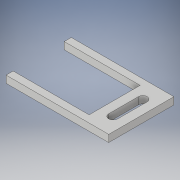
# Autodesk Inventor part: FixScan
Saved by Autodesk Inventor 2017 (Build 210142000, 142)
## iProperties
Part Number: FixScan
Material: Типовые
Document SubType Name: Modeling
Designer: yulia_000
Density: 1 g/cm^3
Appearance: По умолчанию
Author: yulia_000
Autodesk Inventor part; units mm, degrees
ref_plane "YZ Plane" through (0, 0, 0) normal (1, 0, 0) x (0, 1, 0)
ref_plane "XZ Plane" through (0, 0, 0) normal (0, 1, 0) x (-1, 0, 0)
ref_plane "XY Plane" through (0, 0, 0) normal (0, 0, 1) x (1, 0, 0)
sketch "Эскиз1" plane through (0, 0, 0) normal (0, 1, 0) x (-1, 0, 0)
  line L0 (0, 0) -> (9, 0)
  line L1 (9, 0) -> (9, -2.4)
  line L2 (9, -22) -> (0, -22)
  line L3 (0, -22) -> (0, 0)
  line L4 (9, -22) -> (34.6, -22)
  line L5 (34.6, -22) -> (34.6, -19.6)
  line L6 (34.6, -19.6) -> (9, -19.6)
  line L7 (9, -11) -> (0, -11)
  line L8 (9, 0) -> (34.6, 0)
  line L9 (34.6, 0) -> (34.6, -2.4)
  line L10 (34.6, -2.4) -> (9, -2.4)
  line L11 (9, -2.4) -> (9, -22)
  line L12 (4.5, -6) -> (4.5, -16) construction
  line L13 (3, -6) -> (3, -16)
  line L14 (6, -16) -> (6, -6)
  arc A0 (6, -6) -> (3, -6) centre (4.5, -6) ccw
  arc A1 (3, -16) -> (6, -16) centre (4.5, -16) ccw
  point P0 (4.5, -11)
  dimension "d0" = 9
  dimension "d1" = 22
  dimension "d2" = 25.6
  dimension "d3" = 2.4
  dimension "d4" = 5
  dimension "d5" = 3
  dimension "d6" = 30.1
  constraints: 32 end point, 4 parallel, 4 perpendicular, 4 point on circle, 4 tangent, 3 midpoint, 3 symmetric about line, 2 centre point, 2 horizontal, 2 point on line, 2 vertical
  measures "d0" distance of L2.start L2.end
  measures "d1" distance of L2.end L0.start
  measures "d2" distance of L2.start L4.end
  measures "d3" distance of L4.end L5.end
  measures "d4" distance of point (4.5, -11) L12.end
  measures "d5" diameter of A1
  measures "d6" distance between parallel lines of L5 L12
extrude "Выдавливание1" add sketch "Эскиз1" along normal blind 2.4 contours L0 L1 L11 L7 L14 A0 L13 L3 | L8 L9 L10 L1 | L7 L13 A1 L14 L11 L2 L3 | L11 L6 L5 L4
